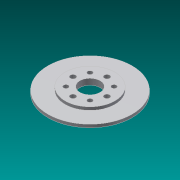
# Autodesk Inventor part: 付け根ロール_サブフレーム_1_4
Saved by Autodesk Inventor 2016 (Build 200138000, 138)
## iProperties
Created: 2016-05-02
Part Number: 付け根ロール_サブフレーム_1_4
Material: アルミニウム 2014-T4
Document SubType Name: Modeling
Designer: hiroaki
Density: 2.8 g/cm^3
Appearance: サテン
Mass: 6.84669 g
Surface Area: 31.3137 cm^2
Volume: 2.44525 cm^3
Author: hiroaki
Autodesk Inventor part; units mm, degrees
ref_plane "YZ Plane" through (0, 0, 0) normal (1, 0, 0) x (0, 1, 0)
ref_plane "XZ Plane" through (0, 0, 0) normal (0, 1, 0) x (-1, 0, 0)
ref_plane "XY Plane" through (0, 0, 0) normal (0, 0, 1) x (1, 0, 0)
derived "付け根ロール_基礎.ipt"
sketch "スケッチ1" plane through (0, 0, 0) normal (0, 0, 1) x (1, 0, 0)
  circle A0 centre (0, 0) radius 5.05
  circle A1 centre (0, -8.5) radius 1.35
  circle A2 centre (0, -8.5) radius 2.5 construction
  circle A3 centre (-5.6569, -5.6569) radius 1.55 construction
  line L0 (-5.6569, -5.6569) -> (0, 0) construction
  line L1 (0, 0) -> (0, -8.5) construction
  line L2 (-4.835, -8.7241) -> (-7.9022, -7.9022) construction
  line L3 (-7.9022, -7.9022) -> (-8.7241, -4.835) construction
  line L4 (-8.7241, -4.835) -> (-6.4787, -2.5896) construction
  line L5 (-6.4787, -2.5896) -> (-3.4115, -3.4115) construction
  line L6 (-3.4115, -3.4115) -> (-2.5896, -6.4787) construction
  line L7 (-2.5896, -6.4787) -> (-4.835, -8.7241) construction
  circle A4 centre (5.6569, -5.6569) radius 1.55 construction
  line L8 (8.7241, -4.835) -> (7.9022, -7.9022) construction
  line L9 (7.9022, -7.9022) -> (4.835, -8.7241) construction
  line L10 (4.835, -8.7241) -> (2.5896, -6.4787) construction
  line L11 (3.4115, -3.4115) -> (6.4787, -2.5896) construction
  line L12 (2.5896, -6.4787) -> (3.4115, -3.4115) construction
  line L13 (6.4787, -2.5896) -> (8.7241, -4.835) construction
  circle A5 centre (8.5, 0) radius 2.5 construction
  circle A6 centre (8.5, 0) radius 1.35
  circle A7 centre (5.6569, 5.6569) radius 1.55 construction
  line L14 (4.835, 8.7241) -> (7.9022, 7.9022) construction
  line L15 (7.9022, 7.9022) -> (8.7241, 4.835) construction
  line L16 (8.7241, 4.835) -> (6.4787, 2.5896) construction
  line L17 (3.4115, 3.4115) -> (2.5896, 6.4787) construction
  line L18 (6.4787, 2.5896) -> (3.4115, 3.4115) construction
  line L19 (2.5896, 6.4787) -> (4.835, 8.7241) construction
  circle A8 centre (0, 8.5) radius 2.5 construction
  circle A9 centre (0, 8.5) radius 1.35
  circle A10 centre (-5.6569, 5.6569) radius 1.55 construction
  line L20 (-8.7241, 4.835) -> (-7.9022, 7.9022) construction
  line L21 (-7.9022, 7.9022) -> (-4.835, 8.7241) construction
  line L22 (-4.835, 8.7241) -> (-2.5896, 6.4787) construction
  line L23 (-3.4115, 3.4115) -> (-6.4787, 2.5896) construction
  line L24 (-2.5896, 6.4787) -> (-3.4115, 3.4115) construction
  line L25 (-6.4787, 2.5896) -> (-8.7241, 4.835) construction
  circle A11 centre (-8.5, 0) radius 2.5 construction
  circle A12 centre (-8.5, 0) radius 1.35
  circle A13 centre (0, 0) radius 12.45 construction
  circle A14 centre (0, 0) radius 21 construction
  circle A15 centre (0, 24.25) radius 3.25 construction
  circle A16 centre (0, 24.25) radius 1.05 construction
  circle A17 centre (-24.25, 0) radius 1.05 construction
  circle A18 centre (0, -24.25) radius 1.05 construction
  circle A19 centre (24.25, 0) radius 1.05 construction
  circle A20 centre (-5.6569, 5.6569) radius 1.2
  circle A21 centre (-5.6569, -5.6569) radius 1.2
  circle A22 centre (5.6569, -5.6569) radius 1.2
  circle A23 centre (5.6569, 5.6569) radius 1.2
  circle A24 centre (0, 0) radius 21
  line L26 (2.75, 25.8377) -> (2.75, 22.6623)
  line L27 (2.75, 22.6623) -> (0, 21.0746)
  line L28 (0, 21.0746) -> (-2.75, 22.6623)
  line L29 (-2.75, 22.6623) -> (-2.75, 25.8377)
  line L30 (-2.75, 25.8377) -> (0, 27.4254)
  line L31 (0, 27.4254) -> (2.75, 25.8377)
  dimension "d8" = 2.4
  dimension "d14" = 360
  dimension "d16" = 42
  measures "d8" diameter of A20
  measures "d16" diameter of A24
extrude "押し出し1" add sketch "スケッチ1" along normal blind 3 contours A24
sketch "スケッチ3" plane through (0, 0, 3) normal (0, 0, 1) x (1, 0, 0)
  circle A0 centre (0, 0) radius 21 projected
  circle A1 centre (0, 0) radius 12.45
  dimension "d19" = 24.9
  constraints: 1 centre point, 1 coincident
  measures "d19" diameter of A1
extrude "押し出し2" cut sketch "スケッチ3" against normal blind 1.5
